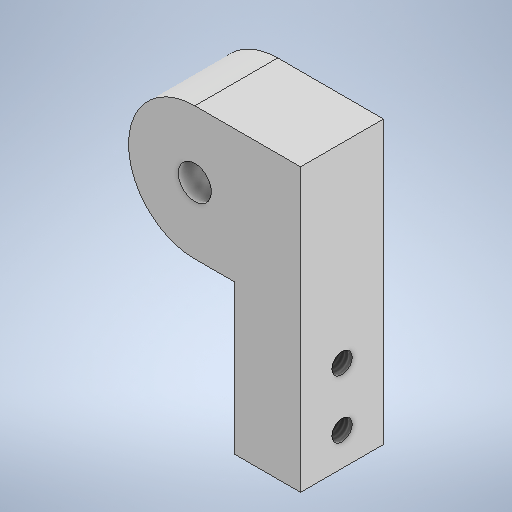
# Autodesk Inventor part: CHUCKLENGAN
Saved by Autodesk Inventor 2025 (Build 290162000, 162)
## iProperties
Created: 2024-12-23
Part Number: CHUCKLENGAN
Material: Generic
Document SubType Name: Modeling
Designer: DMIADX
Density: 1 g/cm^3
Appearance: Default
Author: DMIADX
Autodesk Inventor part; units mm, degrees
ref_plane "YZ Plane" through (0, 0, 0) normal (1, 0, 0) x (0, 1, 0)
ref_plane "XZ Plane" through (0, 0, 0) normal (0, 1, 0) x (-1, 0, 0)
ref_plane "XY Plane" through (0, 0, 0) normal (0, 0, 1) x (1, 0, 0)
sketch "Sketch3" plane through (0, 0, 0) normal (0, 0, 1) x (1, 0, 0)
  circle A0 centre (0, 0) radius 2
  line L0 (0, 0) -> (12.75, 0)
  line L1 (12.75, 0) -> (12.75, -26)
  line L2 (12.75, -26) -> (4.75, -26)
  line L3 (4.75, -26) -> (4.75, -16)
  circle A1 centre (0, 0) radius 12.75
  line L4 (4.75, -16) -> (4.75, 8)
  line L5 (4.75, 8) -> (12.75, 8)
  line L6 (12.75, 8) -> (12.75, 0)
  circle A2 centre (0, 0) radius 8
  line L7 (0, -8) -> (4.75, -8)
  line L8 (0, 8) -> (4.75, 8)
  dimension "d29" = 4
  dimension "d30" = 12.75
  dimension "d31" = 26
  dimension "d32" = 8
  dimension "d33" = 10
  dimension "d34" = 8
  constraints: 18 end point, 6 perpendicular, 3 coincident, 2 centre point, 2 horizontal, 2 point on circle, 1 horizontal alignment, 1 point on line, 1 vertical, 2 other
  measures "d29" diameter of A0
  measures "d30" distance of L0.start L0.end
  measures "d31" distance of L0.end L1.end
  measures "d32" distance of L1.end L2.end
  measures "d33" distance of L2.end L3.end
  measures "d34" distance from line of point (0, 0) L5
extrude "Extrusion2" add sketch "Sketch3" along normal mid plane 10 contours A2 L4 L5 A1 L0 | A2 L4 L0 | L0 L4 A2 | L0 A1 L4 A2 | L1 L2 L3 L4 A1 | A1 L5 L6 | L4 A2 | A2 L8 L4 | L4 L7 A2
sketch "Sketch4" plane through (12.75, -26, 5) normal (1, 0, 0) x (0, 0, -1)
  line L0 (10, 0) -> (0, 0) projected
  point P0 (5, 26)
  point P1 (5, 4)
  point P2 (5, 11)
  dimension "d37" = 7
  dimension "d38" = 4
  measures "d37" distance of point (5, 11) point (5, 4)
  measures "d38" distance from line of L0 point (5, 4)
hole "Hole2" at (12.75, -22, 0) at (12.75, -15, 0) direction (-1, 0, 0) diameter 2.459 end through all thread size "M3x0.5" class "6H" standard "ISO Metric profile"
body "Solid1"
